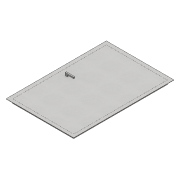
# Autodesk Inventor part: H3NE-D
Saved by Autodesk Inventor 2017 (Build 210142000, 142)
## iProperties
Created: 2016-11-30
Part Number: H3NE-D
Material: Steel, Galvanized
Document SubType Name: Modeling
Designer: krosie
Density: 7.85 g/cm^3
Appearance: Galvanized
Description: Enclosure Door
Author: krosie
Autodesk Inventor part; units mm, degrees
ref_plane "YZ Plane" through (0, 0, 0) normal (1, 0, 0) x (0, 1, 0)
ref_plane "XZ Plane" through (0, 0, 0) normal (0, 1, 0) x (-1, 0, 0)
ref_plane "XY Plane" through (0, 0, 0) normal (0, 0, 1) x (1, 0, 0)
sketch "Sketch1" plane through (0, 0, 0) normal (0, 0, 1) x (1, 0, 0)
  line L0 (-379.8, -583) -> (379.8, -583)
  line L1 (379.8, -583) -> (379.8, 583)
  line L2 (379.8, 583) -> (-379.8, 583)
  line L3 (-379.8, 583) -> (-379.8, -583)
  line L4 (-379.8, -583) -> (379.8, 583) construction
  line L5 (379.8, -583) -> (-379.8, 583) construction
  point P0 (0, 0)
  dimension "d0" = 759.6
  dimension "d1" = 1166
  constraints: 12 end point, 2 midpoint, 2 parallel, 1 horizontal, 1 perpendicular
  measures "d0" distance of L2.end L1.end
  measures "d1" distance of L1.end L0.end
extrude "Extrusion1" add sketch "Sketch1" along normal blind 3
sketch "Sketch2" plane through (0, 0, 3) normal (0, 0, 1) x (1, 0, 0)
  line L0 (379.8, 583) -> (-379.8, 583) projected
  line L1 (379.8, -583) -> (379.8, 583) projected
  line L2 (-379.8, -583) -> (379.8, -583) projected
  line L3 (-379.8, 583) -> (-379.8, -583) projected
  line L4 (-376.8, 580) -> (376.8, 580)
  line L5 (376.8, 580) -> (376.8, -580)
  line L6 (376.8, -580) -> (-376.8, -580)
  line L7 (-376.8, -580) -> (-376.8, 580)
  point P0 (0, 0)
  dimension "d4" = 3
  constraints: 8 end point, 3 other
  measures "d4" distance between parallel lines of L0 L4
extrude "Extrusion2" add sketch "Sketch2" against normal blind 50
sketch "Sketch3" plane through (0, 0, 3) normal (0, 0, 1) x (1, 0, 0)
  line L0 (-299.8, -7.5) -> (-274.8, -7.5)
  line L1 (-274.8, -7.5) -> (-274.8, 7.5)
  line L2 (-274.8, 7.5) -> (-299.8, 7.5)
  line L3 (-299.8, 7.5) -> (-299.8, -7.5)
  line L4 (-299.8, -7.5) -> (-274.8, 7.5) construction
  line L5 (-274.8, -7.5) -> (-299.8, 7.5) construction
  line L6 (-379.8, 583) -> (-379.8, -583) projected
  point P0 (0, 0)
  point P1 (-287.3, 0)
  dimension "d7" = 25
  dimension "d8" = 15
  dimension "d9" = 80
  constraints: 12 end point, 2 midpoint, 2 parallel, 1 horizontal, 1 perpendicular
  measures "d7" distance of L2.end L1.end
  measures "d8" distance of L1.end L0.end
  measures "d9" distance between parallel lines of L6 L3
extrude "Extrusion3" add sketch "Sketch3" along normal blind 35
sketch "Sketch4" plane through (-274.8, -7.5, 3) normal (1, 0, 0) x (0, 0, -1)
  line L0 (-35, 0) -> (-35, 15) projected
  line L1 (-35, 15) -> (-20, 15)
  line L2 (-20, 15) -> (-20, 0)
  line L3 (-20, 0) -> (-35, 0)
  line L4 (-35, 0) -> (-35, 15)
  point P0 (3, 7.5)
  dimension "d12" = 15
  dimension "d13" = 15
  constraints: 8 end point, 2 parallel, 1 horizontal, 1 perpendicular
  measures "d12" distance of L2.end L3.end
  measures "d13" distance of L1.end L2.end
extrude "Extrusion4" add sketch "Sketch4" along normal blind 80
draft "FaceDraft2" angle 1 pull direction (1, 0, 0) faces at (-256.4667, 7.5, 33) fixed edges at (-274.8, 7.5, 13)
sketch "Sketch5" plane through (-379.8, 583, 3) normal (0, 1, 0) x (1, 0, 0)
  line L0 (80, 0) -> (80, -35) construction
  line L1 (105, 0) -> (105, -20) construction
  line L2 (80, 0) -> (105, 0) construction
  line L3 (759.6, 0) -> (0, 0) projected
  line L4 (92.5, 0) -> (92.5, 80) construction
  circle A0 centre (92.5, 40) radius 6
  line L5 (0, 50) -> (759.6, 50) projected
  point P0 (379.8, 3)
  dimension "d18" = 12.5
  dimension "d19" = 12
  dimension "d20" = 10
  constraints: 4 end point, 1 centre point, 1 collinear, 1 midpoint, 1 perpendicular, 1 point on line
  measures "d18" distance between parallel lines of L1 L4
  measures "d19" diameter of A0
  measures "d20" distance from line of A0.centre L5
extrude "Extrusion5" cut sketch "Sketch5" against normal through all
sketch "Sketch7" plane through (0, 0, 3) normal (0, 0, 1) x (1, 0, 0)
  line L0 (379.8, 583) -> (-379.8, 583) projected
  line L1 (-379.8, 583) -> (-379.8, -583) projected
  line L2 (379.8, -583) -> (379.8, 583) projected
  line L3 (-379.8, -583) -> (379.8, -583) projected
  line L4 (-419.8, 623) -> (419.8, 623)
  line L5 (419.8, 623) -> (419.8, -623)
  line L6 (419.8, -623) -> (-419.8, -623)
  line L7 (-419.8, -623) -> (-419.8, 623)
  point P0 (0, 0)
  dimension "d26" = 40
  constraints: 8 end point, 3 other
  measures "d26" distance between parallel lines of L0 L4
extrude "Extrusion7" add sketch "Sketch7" against normal blind 3
body "Solid1"
